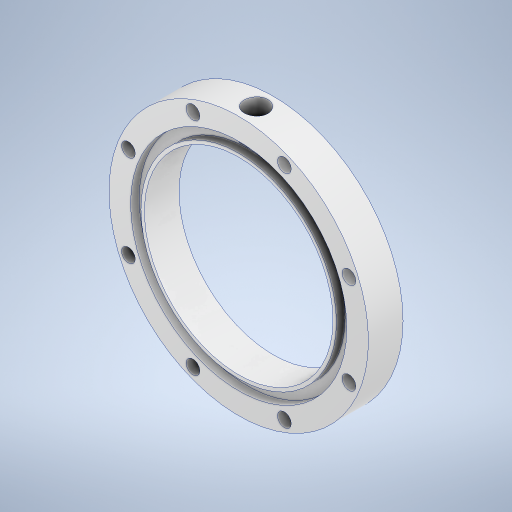
# Autodesk Inventor part: front
Saved by Autodesk Inventor 2023 (Build 270158000, 158)
## iProperties
Created: 2022-09-21
Part Number: front
Material: Aluminum 6061
Document SubType Name: Modeling
Designer: station
Density: 2.7 g/cm^3
Appearance: Aluminum - Flat
Author: station
Autodesk Inventor part; units mm, degrees
ref_plane "YZ Plane" through (0, 0, 0) normal (1, 0, 0) x (0, 1, 0)
ref_plane "XY Plane" through (0, 0, 0) normal (0, 0, 1) x (1, 0, 0)
sketch "Sketch1" plane through (0, 0, 0) normal (0, 0, 1) x (1, 0, 0)
  circle A0 centre (0, 0) radius 54.5
  circle A1 centre (0, 0) radius 75
  circle A2 centre (0, 0) radius 56.5
  circle A3 centre (0, 0) radius 62.5
  circle A4 centre (0, 0) radius 69
  line L0 (0, 0) -> (0, 69) construction
  line L1 (0, 0) -> (26.4052, 63.7477) construction
  line L2 (0, 0) -> (69, 0) construction
  circle A5 centre (26.4052, 63.7477) radius 4
  circle A6 centre (-26.4052, 63.7477) radius 4
  circle A7 centre (-63.7477, 26.4052) radius 4
  circle A8 centre (-63.7477, -26.4052) radius 4
  circle A9 centre (-26.4052, -63.7477) radius 4
  circle A10 centre (26.4052, -63.7477) radius 4
  circle A11 centre (63.7477, -26.4052) radius 4
  circle A12 centre (63.7477, 26.4052) radius 4
  dimension "d0" = 109
  dimension "d1" = 150
  dimension "d2" = 113
  dimension "d3" = 125
  dimension "d4" = 138
  dimension "d16" = 67.5
  dimension "d17" = 8
  dimension "d70" = 360
  constraints: 13 centre point, 6 coincident, 6 end point, 2 point on circle, 1 equal length, 1 horizontal, 1 vertical, 17 other
  measures "d0" diameter of A0
  measures "d1" diameter of A1
  measures "d2" diameter of A2
  measures "d3" diameter of A3
  measures "d4" diameter of A4
  measures "d16" angle of L2 L1
  measures "d17" diameter of A5
extrude "Extrusion1" add sketch "Sketch1" along normal blind 20 contours A2
extrude "Extrusion2" add sketch "Sketch1" along normal blind 15 contours A3
extrude "Extrusion3" add sketch "Sketch1" along normal blind 20 contours A1 | A4 A11 A10 A9 A8 A7 A6 A5 A12 | A12 A4 | A4 A12 | A11 A4 | A4 A11 | A5 A4 | A4 A5 | A10 A4 | A4 A10 | A6 A4 | A4 A6 | A9 A4 | A4 A9 | A7 A4 | A4 A7 | A8 A4 | A4 A8
ref_plane "Work Plane1" through (0, 75, 0) normal (0, 1, 0) x (-1, 0, 0)
sketch "Sketch2" plane through (0, 75, 0) normal (0, 1, 0) x (-1, 0, 0)
  line L0 (0, 0) -> (0, 10) construction
  circle A0 centre (0, 10) radius 6.858
  dimension "d12" = 10
  dimension "d13" = 13.716
  constraints: 2 end point, 1 centre point, 1 coincident, 1 vertical
  measures "d12" distance of L0.start L0.end
  measures "d13" diameter of A0
extrude "Extrusion4" cut sketch "Sketch2" against normal blind 18
hole "Hole1" at (26.4052, 63.7477, 0) at (63.7477, 26.4052, 0) at (63.7477, -26.4052, 0) at (26.4052, -63.7477, 0) at (-26.4052, -63.7477, 0) at (-63.7477, -26.4052, 0) at (-26.4052, 63.7477, 0) at (-63.7477, 26.4052, 0) direction (0, 0, 1) diameter 8 end through all
body "Solid1"
